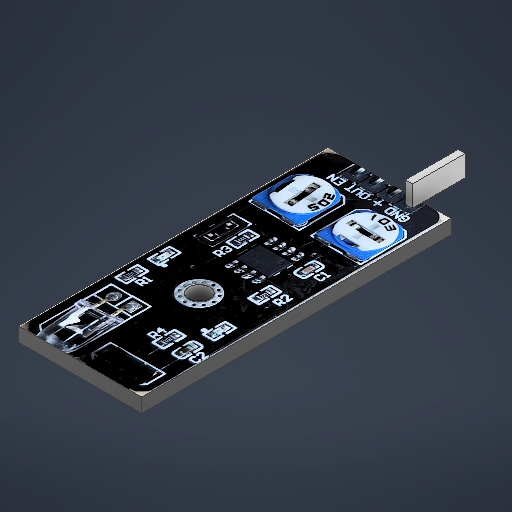
# Autodesk Inventor part: 3DModel
Saved by Autodesk Inventor 2026.2 (Build 302298000, 298)
## iProperties
Created: 2025-06-04
Part Number: 3DModel
Material: Generic
Document SubType Name: Modeling
Designer: cdavi
Density: 1 g/cm^3
Appearance: Default
Mass: 1.52586 g
Surface Area: 17.9071 cm^2
Volume: 1.52586 cm^3
Author: cdavi
Autodesk Inventor part; units mm, degrees
ref_plane "YZ Plane" through (0, 0, 0) normal (1, 0, 0) x (0, 1, 0)
ref_plane "XZ Plane" through (0, 0, 0) normal (0, 1, 0) x (-1, 0, 0)
ref_plane "XY Plane" through (0, 0, 0) normal (0, 0, 1) x (1, 0, 0)
sketch "Sketch1" plane through (0, 0, 0) normal (0, 1, 0) x (-1, 0, 0)
  line L0 (-8.75, 22) -> (-8.75, -22)
  line L1 (-8.75, -22) -> (8.75, -22)
  line L2 (8.75, -22) -> (8.75, 22)
  line L3 (8.75, 22) -> (-8.75, 22)
  line L4 (-8.75, 22) -> (8.75, -22) construction
  line L5 (-8.75, -22) -> (8.75, 22) construction
  line L6 (-8.75, 22) -> (-1.75, 22)
  point P0 (0, 0)
  dimension "d1" = 44
  dimension "d2" = 17.5
  constraints: 14 end point, 2 midpoint, 2 parallel, 1 horizontal, 1 perpendicular, 1 vertical
  measures "d1" distance of L1.end L2.end
  measures "d2" distance of L0.end L1.end
extrude "Extrusion1" add sketch "Sketch1" along normal blind 2
sketch "Sketch2" plane through (0, 2, 0) normal (0, 1, 0) x (1, 0, 0)
  line L0 (8.75, 22) -> (-8.75, 22) projected
  line L1 (-8.6195, 22) -> (8.6907, 22) construction
  line L2 (8.6907, 22) -> (8.6907, -23.9682) construction
  line L3 (8.6907, -23.9682) -> (-8.6195, -23.9682) construction
  line L4 (-8.6195, -23.9682) -> (-8.6195, 22) construction
  circle A0 centre (0.05, -5.1) radius 1.5
  line L5 (8.75, -22) -> (8.75, 22) projected
  line L6 (-8.75, -22) -> (8.75, -22) projected
  point P0 (0, 0)
  dimension "d39" = 3
  dimension "d42" = 8.7
  dimension "d43" = 16.9
  constraints: 1 centre point, 1 point on line, 1 vertical, 2 other
  measures "d39" diameter of A0
  measures "d42" distance from line of A0.centre L5
  measures "d43" distance from line of L6 A0.centre
decal "Decal1"
sketch "Sketch3" plane through (0, 2, 0) normal (0, 1, 0) x (1, 0, 0)
  circle A0 centre (0.05, -5.1) radius 1.5
  line L0 (8.75, -22) -> (8.75, -101.371)
  line L1 (-21.6488, -22) -> (8.75, -22)
  line L2 (8.75, -22) -> (8.75, 22) projected
  line L3 (-8.75, -22) -> (8.75, -22) projected
  point P0 (0, 0)
  point P1 (-12.8988, -61.6855)
  dimension "d44" = 3
  dimension "d45" = 8.7
  dimension "d46" = 16.9
  constraints: 4 end point, 2 collinear, 1 centre point
  measures "d44" diameter of A0
  measures "d45" distance from line of A0.centre L0
  measures "d46" distance from line of L1 A0.centre
extrude "Extrusion2" cut sketch "Sketch3" against normal through all
sketch "Sketch4" plane through (0, 2, 0) normal (0, 1, 0) x (1, 0, 0)
  line L0 (4.75, 20.5) -> (3.75, 20.5)
  line L1 (3.75, 20.5) -> (3.75, 28)
  line L2 (3.75, 28) -> (4.75, 28)
  line L3 (4.75, 28) -> (4.75, 20.5)
  line L4 (8.75, -22) -> (8.75, 22) projected
  line L5 (8.75, 22) -> (-8.75, 22) projected
  point P0 (0, 0)
  dimension "d51" = 4
  dimension "d52" = 1
  dimension "d53" = 1.5
  dimension "d54" = 7.5
  constraints: 8 end point, 2 parallel, 1 horizontal, 1 perpendicular
  measures "d51" distance between parallel lines of L3 L4
  measures "d52" distance between parallel lines of L3 L1
  measures "d53" distance between parallel lines of L5 L0
  measures "d54" distance of L0.end L1.end
extrude "Extrusion3" add sketch "Sketch4" along normal blind 3
body "Solid1"
